45 teeth 18 hole (Autodesk Fusion 360 design; units mm, degrees)
description: Spur Gear; Module: 1.27; Num Teeth: 45; Pressure Angle: 20.0; Backlash: 0.00 mm
part number: 2026-06-12-02-46-04-077
Autodesk Fusion 360 part; units mm, degrees
sketch "Base Circle" plane through (0, 0, 0) normal (0, 0, 1) x (1, 0, 0)
  circle A0 centre (0, 0) radius 27.1056
  circle A1 centre (0, 0) radius 9
extrude "Extrude1" add sketch "Base Circle" along normal blind 1
sketch "Gear Tooth" plane through (0, 0, 0) normal (0, 0, 1) x (1, 0, 0)
  spline S0 degree 5 poles (26.8184, -1.337) (26.8271, -1.337) (26.8445, -1.337) (26.8706, -1.3368) (26.9054, -1.3362) (26.9489, -1.3346) (26.9925, -1.3324) (27.036, -1.3295) (27.0796, -1.3259) (27.1232, -1.3218) (27.1667, -1.3171) (27.2103, -1.3119) (27.2539, -1.3063) (27.2974, -1.3003) (27.341, -1.294) (27.3845, -1.2874) (27.4281, -1.2804) (27.4716, -1.273) (27.5152, -1.2653) (27.5587, -1.2573) (27.6022, -1.249) (27.6457, -1.2403) (27.6892, -1.2313) (27.7327, -1.2221) (27.7762, -1.2126) (27.8196, -1.2028) (27.8631, -1.1927) (27.9065, -1.1824) (27.9499, -1.1718) (27.9933, -1.1609) (28.0367, -1.1498) (28.0801, -1.1384) (28.1235, -1.1268) (28.1668, -1.115) (28.2101, -1.1029) (28.2534, -1.0905) (28.2967, -1.0779) (28.34, -1.0651) (28.3833, -1.0521) (28.4265, -1.0389) (28.4697, -1.0254) (28.513, -1.0117) (28.5561, -0.9978) (28.5993, -0.9837) (28.6424, -0.9693) (28.6856, -0.9548) (28.7287, -0.94) (28.7718, -0.925) (28.8148, -0.9099) (28.8579, -0.8945) (28.9009, -0.8789) (28.9439, -0.8631) (28.9868, -0.8471) (29.0298, -0.831) (29.0727, -0.8146) (29.1156, -0.798) (29.1585, -0.7813) (29.2013, -0.7643) (29.2442, -0.7472) (29.287, -0.7299) (29.3298, -0.7124) (29.3725, -0.6947) (29.4152, -0.6768) (29.4579, -0.6588) (29.5006, -0.6405) (29.5433, -0.6221) (29.5859, -0.6035) (29.6285, -0.5847) (29.671, -0.5658) (29.7136, -0.5466) (29.7561, -0.5273) (29.7901, -0.5118) (29.8155, -0.5) (29.8325, -0.4921) (29.841, -0.4882) knots 0 0 0 0 0 0 0.01428571 0.02857143 0.04285714 0.05714286 0.07142857 0.08571429 0.1 0.11428571 0.12857143 0.14285714 0.15714286 0.17142857 0.18571429 0.2 0.21428571 0.22857143 0.24285714 0.25714286 0.27142857 0.28571429 0.3 0.31428571 0.32857143 0.34285714 0.35714286 0.37142857 0.38571429 0.4 0.41428571 0.42857143 0.44285714 0.45714286 0.47142857 0.48571429 0.5 0.51428571 0.52857143 0.54285714 0.55714286 0.57142857 0.58571429 0.6 0.61428571 0.62857143 0.64285714 0.65714286 0.67142857 0.68571429 0.7 0.71428571 0.72857143 0.74285714 0.75714286 0.77142857 0.78571429 0.8 0.81428571 0.82857143 0.84285714 0.85714286 0.87142857 0.88571429 0.9 0.91428571 0.92857143 0.94285714 0.95714286 0.97142857 0.98571429 1 1 1 1 1 1
  spline S1 degree 5 poles (26.8184, 1.337) (26.8271, 1.337) (26.8445, 1.337) (26.8706, 1.3368) (26.9054, 1.3362) (26.9489, 1.3346) (26.9925, 1.3324) (27.036, 1.3295) (27.0796, 1.3259) (27.1232, 1.3218) (27.1667, 1.3171) (27.2103, 1.3119) (27.2539, 1.3063) (27.2974, 1.3003) (27.341, 1.294) (27.3845, 1.2874) (27.4281, 1.2804) (27.4716, 1.273) (27.5152, 1.2653) (27.5587, 1.2573) (27.6022, 1.249) (27.6457, 1.2403) (27.6892, 1.2313) (27.7327, 1.2221) (27.7762, 1.2126) (27.8196, 1.2028) (27.8631, 1.1927) (27.9065, 1.1824) (27.9499, 1.1718) (27.9933, 1.1609) (28.0367, 1.1498) (28.0801, 1.1384) (28.1235, 1.1268) (28.1668, 1.115) (28.2101, 1.1029) (28.2534, 1.0905) (28.2967, 1.0779) (28.34, 1.0651) (28.3833, 1.0521) (28.4265, 1.0389) (28.4697, 1.0254) (28.513, 1.0117) (28.5561, 0.9978) (28.5993, 0.9837) (28.6424, 0.9693) (28.6856, 0.9548) (28.7287, 0.94) (28.7718, 0.925) (28.8148, 0.9099) (28.8579, 0.8945) (28.9009, 0.8789) (28.9439, 0.8631) (28.9868, 0.8471) (29.0298, 0.831) (29.0727, 0.8146) (29.1156, 0.798) (29.1585, 0.7813) (29.2013, 0.7643) (29.2442, 0.7472) (29.287, 0.7299) (29.3298, 0.7124) (29.3725, 0.6947) (29.4152, 0.6768) (29.4579, 0.6588) (29.5006, 0.6405) (29.5433, 0.6221) (29.5859, 0.6035) (29.6285, 0.5847) (29.671, 0.5658) (29.7136, 0.5466) (29.7561, 0.5273) (29.7901, 0.5118) (29.8155, 0.5) (29.8325, 0.4921) (29.841, 0.4882) knots 0 0 0 0 0 0 0.01428571 0.02857143 0.04285714 0.05714286 0.07142857 0.08571429 0.1 0.11428571 0.12857143 0.14285714 0.15714286 0.17142857 0.18571429 0.2 0.21428571 0.22857143 0.24285714 0.25714286 0.27142857 0.28571429 0.3 0.31428571 0.32857143 0.34285714 0.35714286 0.37142857 0.38571429 0.4 0.41428571 0.42857143 0.44285714 0.45714286 0.47142857 0.48571429 0.5 0.51428571 0.52857143 0.54285714 0.55714286 0.57142857 0.58571429 0.6 0.61428571 0.62857143 0.64285714 0.65714286 0.67142857 0.68571429 0.7 0.71428571 0.72857143 0.74285714 0.75714286 0.77142857 0.78571429 0.8 0.81428571 0.82857143 0.84285714 0.85714286 0.87142857 0.88571429 0.9 0.91428571 0.92857143 0.94285714 0.95714286 0.97142857 0.98571429 1 1 1 1 1 1
  arc A0 (29.841, -0.4882) -> (29.841, 0.4882) centre (0, 0) ccw
  line L0 (26.8184, 1.337) -> (26.8184, -1.337)
  point P0 (27.0328, -1.3296)
  point P1 (27.248, -1.307)
  point P2 (27.4636, -1.2743)
  point P3 (27.6795, -1.2333)
  point P4 (27.8956, -1.1849)
  point P5 (28.1119, -1.1299)
  point P6 (28.3282, -1.0686)
  point P7 (28.5446, -1.0015)
  point P8 (28.761, -0.9287)
  point P9 (28.9773, -0.8507)
  point P10 (29.1935, -0.7674)
  point P11 (29.4095, -0.6792)
  point P12 (29.6254, -0.586)
  point P13 (27.0328, 1.3296)
  point P14 (27.248, 1.307)
  point P15 (27.4636, 1.2743)
  point P16 (27.6795, 1.2333)
  point P17 (27.8956, 1.1849)
  point P18 (28.1119, 1.1299)
  point P19 (28.3282, 1.0686)
  point P20 (28.5446, 1.0015)
  point P21 (28.761, 0.9287)
  point P22 (28.9773, 0.8507)
  point P23 (29.1935, 0.7674)
  point P24 (29.4095, 0.6792)
  point P25 (29.6254, 0.586)
extrude "Extrude2" add sketch "Gear Tooth" along normal blind 1
fillet "Fillet1" radius 0.2 2 edges at (27.0731, 1.3263, 0.5) (27.0731, -1.3263, 0.5)
pattern_circular "C-Pattern1" count 45 over 360 about axis through (0, 0, 0) along (0, 0, 1) of "Extrude2", "Fillet1"
sketch "Diametrial Pitch Circle" plane through (0, 0, 0) normal (0, 0, 1) x (1, 0, 0)
  circle A0 centre (0, 0) radius 28.575 construction
extrude "Extrude3" add 1 faces at (-10.5214, -18.2237, 0) along direction (0, 0, -1) blind 2
named bodies: "Spur Gear (45 teeth)"
